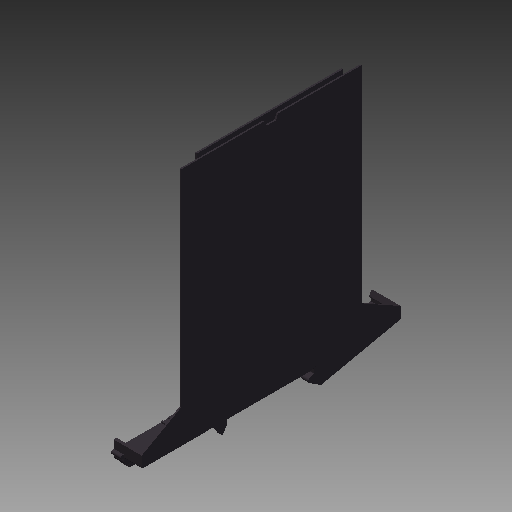
# Autodesk Inventor part: CH20M22 B R BK 2410160000
Saved by Autodesk Inventor 2019.3 (Build 233278000, 278)
## iProperties
Category: PARTsolutions
Company: WEIDMUELLER
Created: 2018-11-15
Part Number: CH20M22 B R BK 2410160000
Material: Generic
Catalog Web Link: www.cadenas.de
Description: CH20M22 B RE-CH20M
Vendor: WEIDMUELLER
Document SubType Name: Modeling
Designer: psadmin
Manufacturer: WEIDMUELLER
Mass: 10.5122 g
Surface Area: 188.227 cm^2
Volume: 10.5122 cm^3
Density: 1 g/cm^3
Appearance: PSOLRGB-68-61-68
PSOL_IDENT_0: {$CADENAS_DATA\23d-libs\weidmueller\elektronikgehaeuse\einbaugehaeuse\ch20m\einzelteile\ch20m22-5\ch
PSOL_IDENT_1: 20m22-b-re.prj},196 {VTYP=3D},{NB=CH20M22 B R BK 2410160000},{LINA=CH20M22 B R BK 2410160000},{NN=CH
PSOL_IDENT_2: 20M22 B RE},{DATE=18.01.2013 16:41:43},{GEOMDATE=29.10.2012 09:45:00},{VERSION=},{LINEID=60},{WBVAR=
PSOL_IDENT_3: },{WBNUMERIC=}  {NB=CH20M22 B R BK 2410160000},{LINA=CH20M22 B R BK 2410160000},{KT=DUMMY},{BEST=241
PSOL_IDENT_4: 0160000},{BZ=CH20M22 B R BK},{F=schwarz},{FCODE=0.27,0.24,0.27,0.00},{VAR=1}
NN: CH20M22 B RE
NT: CH20M
NB: CH20M22 B R BK 2410160000
NBSYN: $BZ. $BEST.
LINA: CH20M22 B R BK 2410160000
BEST: 2410160000
BZ: CH20M22 B R BK
F: black
VAR: 1
SUPPLIER: WEIDMUELLER
ARTICLENO: CH20M22 B R BK 2410160000
BOMINFO: CH20M22 B R BK 2410160000
CREATOR: CADENAS GmbH
Title: CH20M22 B R BK 2410160000
Author: Cadenas PARTsolutions
Comments: CH20M
Autodesk Inventor part; units mm, degrees
sketch "Sketch_3" plane through (11.25, 0, 0) normal (1, 0, 0) x (0, 0, -1)
  line L0 (-52.8502, 4.6704) -> (-52.8502, 0.4996)
  arc A0 (-52.8502, 0.4996) -> (-52.3502, -0.0004) centre (-52.3502, 0.4996) ccw
  line L1 (-52.3502, -0.0004) -> (-26.1677, -0.0004)
  line L2 (-26.1677, -0.0004) -> (-26.1678, 0.2671)
  arc A1 (-25.666, 0.7668) -> (-26.1678, 0.2671) centre (-25.6671, 0.2661) ccw
  line L3 (-25.666, 0.7668) -> (15.1495, 0.7669)
  arc A2 (15.1495, 0.7669) -> (15.5941, 0.8453) centre (15.1495, 2.0669) ccw
  line L4 (15.5941, 0.8453) -> (16.5371, 1.1885)
  arc A3 (18.2817, -0.0331) -> (16.5371, 1.1885) centre (16.9817, -0.0331) ccw
  line L5 (18.2817, -0.0331) -> (18.2817, -2.0061)
  arc A4 (18.1501, -2.1941) -> (18.2817, -2.0061) centre (18.0817, -2.0061) ccw
  line L6 (18.1501, -2.1941) -> (16.1263, -2.9307)
  arc A5 (16.1263, -2.9307) -> (16.084, -3.2852) centre (16.1947, -3.1186) ccw
  line L7 (16.084, -3.2852) -> (20.3709, -6.1333)
  arc A6 (20.3709, -6.1333) -> (20.5236, -6.1623) centre (20.4815, -5.9667) ccw
  line L8 (20.5236, -6.1623) -> (52.8497, 0.7929)
  line L9 (52.8497, 0.7929) -> (52.8497, 4.6323)
  line L10 (52.8497, 4.6323) -> (36.8, 13.6205)
  line L11 (36.8, 13.6205) -> (36.8, 97.7)
  line L12 (36.8, 97.7) -> (2.9593, 97.7)
  arc A7 (2.9593, 97.7) -> (2.7327, 97.5557) centre (2.9593, 97.45) ccw
  line L13 (2.7327, 97.5557) -> (1.9347, 95.8443)
  arc A8 (1.7081, 95.7) -> (1.9347, 95.8443) centre (1.7081, 95.95) ccw
  line L14 (1.7081, 95.7) -> (-1.7081, 95.7)
  arc A9 (-1.9347, 95.8443) -> (-1.7081, 95.7) centre (-1.7081, 95.95) ccw
  line L15 (-1.9347, 95.8443) -> (-2.7327, 97.5557)
  arc A10 (-2.7327, 97.5557) -> (-2.9593, 97.7) centre (-2.9593, 97.45) ccw
  line L16 (-2.9593, 97.7) -> (-36.8, 97.7)
  line L17 (-36.8, 97.7) -> (-36.8, 13.6589)
  line L18 (-36.8, 13.6589) -> (-52.8502, 4.6704)
  constraints: 38 end point, 22 point on circle, 11 centre point
extrude "Extrusion1" add sketch "Sketch_3" against normal blind 0.6
sketch "Sketch_4" plane through (0, 0, 0) normal (1, 0, 0) x (0, 1, 0)
  line L0 (4.6704, 52.8502) -> (0.4996, 52.8502)
  arc A0 (0.4996, 52.8502) -> (-0.0004, 52.3502) centre (0.4996, 52.3502) ccw
  line L1 (-0.0004, 52.3502) -> (-0.0004, 26.1677)
  line L2 (-0.0004, 26.1677) -> (0.2671, 26.1678)
  arc A1 (0.7668, 25.666) -> (0.2671, 26.1678) centre (0.2661, 25.6671) ccw
  line L3 (0.7668, 25.666) -> (0.7669, -15.1495)
  arc A2 (0.7669, -15.1495) -> (0.8453, -15.5941) centre (2.0669, -15.1495) ccw
  line L4 (0.8453, -15.5941) -> (1.1885, -16.5371)
  arc A3 (-0.0331, -18.2817) -> (1.1885, -16.5371) centre (-0.0331, -16.9817) ccw
  line L5 (-0.0331, -18.2817) -> (-2.0061, -18.2817)
  arc A4 (-2.1941, -18.1501) -> (-2.0061, -18.2817) centre (-2.0061, -18.0817) ccw
  line L6 (-2.1941, -18.1501) -> (-2.9307, -16.1263)
  arc A5 (-2.9307, -16.1263) -> (-3.2852, -16.084) centre (-3.1186, -16.1947) ccw
  line L7 (-3.2852, -16.084) -> (-6.1333, -20.3709)
  arc A6 (-6.1333, -20.3709) -> (-6.1623, -20.5236) centre (-5.9667, -20.4815) ccw
  line L8 (-6.1623, -20.5236) -> (0.7929, -52.8497)
  line L9 (0.7929, -52.8497) -> (4.6323, -52.8497)
  line L10 (4.6323, -52.8497) -> (5.1117, -51.9936)
  line L11 (5.1117, -51.9936) -> (3.3706, -51.1817)
  line L12 (3.3706, -51.1817) -> (3.0706, -51.1817)
  arc A7 (3.0706, -51.1817) -> (2.9206, -51.3317) centre (3.0706, -51.3317) ccw
  line L13 (2.9206, -51.3317) -> (2.9206, -51.7817)
  line L14 (2.9206, -51.7817) -> (1.2669, -51.7817)
  line L15 (1.2669, -51.7817) -> (1.2669, -50.774)
  line L16 (1.2669, -50.774) -> (-0.1649, -44.1193)
  arc A8 (0.1221, -43.6489) -> (-0.1649, -44.1193) centre (0.2262, -44.0352) ccw
  arc A9 (0.1221, -43.6489) -> (-0.5291, -40.6223) centre (-0.2813, -42.1523) ccw
  arc A10 (-0.9842, -40.3116) -> (-0.5291, -40.6223) centre (-0.5931, -40.2274) ccw
  line L17 (-0.9842, -40.3116) -> (-4.705, -23.0181)
  arc A11 (-4.3238, -22.5341) -> (-4.705, -23.0181) centre (-4.3139, -22.9339) ccw
  arc A12 (-4.3238, -22.5341) -> (-3.6869, -19.1722) centre (-4.3672, -20.7846) ccw
  arc A13 (-3.8645, -18.5824) -> (-3.6869, -19.1722) centre (-3.5314, -18.8037) ccw
  line L18 (-3.8645, -18.5824) -> (-3.4366, -17.9382)
  arc A14 (-3.2593, -17.9594) -> (-3.4366, -17.9382) centre (-3.3533, -17.9936) ccw
  line L19 (-3.2593, -17.9594) -> (-2.8863, -18.9843)
  arc A15 (-2.8863, -18.9843) -> (-2.6044, -19.1817) centre (-2.6044, -18.8817) ccw
  line L20 (-2.6044, -19.1817) -> (-0.0331, -19.1817)
  arc A16 (-0.0331, -19.1817) -> (2.0342, -16.2292) centre (-0.0331, -16.9817) ccw
  line L21 (2.0342, -16.2292) -> (1.6729, -15.2366)
  arc A17 (1.6669, -15.2024) -> (1.6729, -15.2366) centre (1.7669, -15.2024) ccw
  line L22 (1.6669, -15.2024) -> (1.6669, 31.0449)
  line L23 (1.6669, 31.0449) -> (1.3287, 31.0449)
  line L24 (1.3287, 31.0449) -> (1.3287, 33.1213)
  line L25 (1.3287, 33.1213) -> (1.6669, 33.1213)
  line L26 (1.6669, 33.1213) -> (1.6669, 33.8183)
  line L27 (1.6669, 33.8183) -> (1.2169, 33.8183)
  line L28 (1.2169, 33.8183) -> (1.2169, 51.8503)
  line L29 (1.2169, 51.8503) -> (2.9206, 51.8503)
  line L30 (2.9206, 51.8503) -> (2.9206, 51.4003)
  arc A18 (2.9206, 51.4003) -> (3.0706, 51.2503) centre (3.0706, 51.4003) ccw
  line L31 (3.0706, 51.2503) -> (3.3706, 51.2503)
  line L32 (3.3706, 51.2503) -> (5.1117, 52.0622)
  line L33 (5.1117, 52.0622) -> (4.6704, 52.8502)
  constraints: 68 end point, 38 point on circle, 19 centre point
extrude "Extrusion2" add sketch "Sketch_4" along normal blind 10.65
sketch "Sketch_5" plane through (11.15, 0, 0) normal (1, 0, 0) x (0, 0, -1)
  line L0 (-26.1678, 0.2671) -> (-26.1677, -0.0004)
  line L1 (-26.1677, -0.0004) -> (15.3805, -0.0004)
  arc A0 (15.3805, -0.0004) -> (15.8251, 0.078) centre (15.3805, 1.2996) ccw
  line L2 (15.8251, 0.078) -> (16.8107, 0.4368)
  arc A1 (17.4817, -0.0331) -> (16.8107, 0.4368) centre (16.9817, -0.0331) ccw
  line L3 (17.4817, -0.0331) -> (17.4817, -1.446)
  arc A2 (17.3501, -1.6339) -> (17.4817, -1.446) centre (17.2817, -1.446) ccw
  line L4 (17.3501, -1.6339) -> (15.6666, -2.2466)
  arc A3 (15.6666, -2.2466) -> (15.4764, -3.842) centre (15.9744, -3.0924) ccw
  line L5 (15.4764, -3.842) -> (20.2092, -6.9864)
  arc A4 (20.2092, -6.9864) -> (20.362, -7.0153) centre (20.3199, -6.8198) ccw
  line L6 (20.362, -7.0153) -> (52.8497, -0.0254)
  line L7 (52.8497, -0.0254) -> (52.8497, 0.7929)
  line L8 (52.8497, 0.7929) -> (20.5236, -6.1623)
  arc A5 (20.3709, -6.1333) -> (20.5236, -6.1623) centre (20.4815, -5.9667) ccw
  line L9 (20.3709, -6.1333) -> (16.084, -3.2852)
  arc A6 (16.1263, -2.9307) -> (16.084, -3.2852) centre (16.1947, -3.1186) ccw
  line L10 (16.1263, -2.9307) -> (18.1501, -2.1941)
  arc A7 (18.1501, -2.1941) -> (18.2817, -2.0061) centre (18.0817, -2.0061) ccw
  line L11 (18.2817, -2.0061) -> (18.2817, -0.0331)
  arc A8 (18.2817, -0.0331) -> (16.5371, 1.1885) centre (16.9817, -0.0331) ccw
  line L12 (16.5371, 1.1885) -> (15.5444, 0.8272)
  arc A9 (15.2024, 0.7669) -> (15.5444, 0.8272) centre (15.2024, 1.7669) ccw
  line L13 (15.2024, 0.7669) -> (-25.666, 0.7668)
  arc A10 (-25.666, 0.7668) -> (-26.1678, 0.2671) centre (-25.6671, 0.2661) ccw
  constraints: 28 end point, 22 point on circle, 11 centre point
extrude "Extrusion3" add sketch "Sketch_5" against normal blind 2.95
sketch "Sketch_6" plane through (11.15, 0, 0) normal (1, 0, 0) x (0, 0, -1)
  line L0 (-23.8572, 0.7669) -> (-20.2696, -4.3568)
  arc A0 (-20.2696, -4.3568) -> (-19.427, -4.32) centre (-19.86, -4.07) ccw
  line L1 (-19.427, -4.32) -> (-17.934, -1.734)
  arc A1 (-17.934, -1.734) -> (-17.8, -1.234) centre (-18.8, -1.234) ccw
  line L2 (-17.8, -1.234) -> (-17.8, 0.7669)
  line L3 (-17.8, 0.7669) -> (-23.8572, 0.7669)
  constraints: 8 end point, 4 point on circle, 2 centre point
extrude "Extrusion4" add sketch "Sketch_6" against normal blind 1.4
sketch "Sketch_7" plane through (10.65, 0, 0) normal (1, 0, 0) x (0, 0, -1)
  line L0 (-33.8, 6.0553) -> (-33.8, 0.7669)
  line L1 (-33.8, 0.7669) -> (15.1495, 0.7669)
  arc A0 (15.1495, 0.7669) -> (15.5941, 0.8453) centre (15.1495, 2.0669) ccw
  line L2 (15.5941, 0.8453) -> (16.5371, 1.1885)
  arc A1 (18.2817, -0.0331) -> (16.5371, 1.1885) centre (16.9817, -0.0331) ccw
  line L3 (18.2817, -0.0331) -> (18.2817, -2.0061)
  arc A2 (18.1501, -2.1941) -> (18.2817, -2.0061) centre (18.0817, -2.0061) ccw
  line L4 (18.1501, -2.1941) -> (16.1263, -2.9307)
  arc A3 (16.1263, -2.9307) -> (16.084, -3.2852) centre (16.1947, -3.1186) ccw
  line L5 (16.084, -3.2852) -> (20.3709, -6.1333)
  arc A4 (20.3709, -6.1333) -> (20.5236, -6.1623) centre (20.4815, -5.9667) ccw
  line L6 (20.5236, -6.1623) -> (52.8497, 0.7929)
  line L7 (52.8497, 0.7929) -> (52.8497, 1.3)
  line L8 (52.8497, 1.3) -> (33.8, 1.3)
  line L9 (33.8, 1.3) -> (33.8, 6.0169)
  line L10 (33.8, 6.0169) -> (29.8, 8.257)
  line L11 (29.8, 8.257) -> (29.8, 99.5)
  line L12 (29.8, 99.5) -> (-29.8, 99.5)
  line L13 (-29.8, 99.5) -> (-29.8, 8.2954)
  line L14 (-29.8, 8.2954) -> (-33.8, 6.0553)
  constraints: 30 end point, 10 point on circle, 5 centre point
extrude "Extrusion5" add sketch "Sketch_7" against normal blind 0.65
sketch "Sketch_8" plane through (0, 0, 0) normal (1, 0, 0) x (0, 1, 0)
  arc A0 (1.4669, 53.3505) -> (-0.0331, 53.3505) centre (0.7169, 53.3505) ccw
  line L0 (-0.0331, 53.3505) -> (-0.0331, 53.0505)
  arc A1 (-0.2331, 52.8505) -> (-0.0331, 53.0505) centre (-0.2331, 53.0505) ccw
  line L1 (-0.2331, 52.8505) -> (-1.1331, 52.8505)
  arc A2 (-1.1331, 52.8505) -> (-2.7829, 51.2228) centre (-1.1331, 51.2005) ccw
  line L2 (-2.7829, 51.2228) -> (-2.7925, 50.5132)
  line L3 (-2.7925, 50.5132) -> (-4.3007, 50.5132)
  line L4 (-4.3007, 50.5132) -> (-4.3007, 27.5678)
  line L5 (-4.3007, 27.5678) -> (-0.0004, 27.5678)
  line L6 (-0.0004, 27.5678) -> (-0.0004, 51.8503)
  line L7 (-0.0004, 51.8503) -> (1.4669, 51.8503)
  line L8 (1.4669, 51.8503) -> (1.4669, 53.3505)
  constraints: 18 end point, 6 point on circle, 3 centre point
extrude "Extrusion6" add sketch "Sketch_8" along normal blind 4
sketch "Sketch_9" plane through (10, 0, 0) normal (1, 0, 0) x (0, 0, -1)
  line L0 (17.2, 4.5) -> (17.2, 1.5)
  line L1 (17.2, 1.5) -> (18.2, 1.5)
  line L2 (18.2, 1.5) -> (18.2, 4.5)
  arc A0 (18.2, 4.5) -> (17.2, 4.5) centre (17.7, 4.5) ccw
  constraints: 6 end point, 2 point on circle, 1 centre point
extrude "Extrusion7" add sketch "Sketch_9" against normal blind 6.6
ref_plane "CP_XY" through (0, 0, 0) normal (1, 0, 0) x (0, 0, -1)
ref_plane "CP_YZ" through (0, 0, 0) normal (0, 0, -1) x (0, 1, 0)
ref_plane "CP_ZX" through (0, 0, 0) normal (0, 1, 0) x (1, 0, 0)
body "Solid1"
